Autodesk Fusion 360 part; units mm, degrees
(part 3 of 3)
sketch "Sketch2" plane through (0, 0, 0) normal (0, 0, 1) x (1, 0, 0)
  line L0 (0, 75.1711) -> (0, -79.242) construction
  circle A0 centre (30, 30) radius 2
  circle A1 centre (30, -30) radius 2
  circle A2 centre (15.25, 15.25) radius 1.6
  circle A3 centre (15.25, -15.25) radius 1.6
  circle A4 centre (0, -23) radius 6.5
  circle A5 centre (15.25, -31.25) radius 1.6
  line L1 (0, 0) -> (20.75, 0) construction
  line L2 (38.1, 30) -> (0, 30) construction
  circle A6 centre (30, 30) radius 8
  line L3 (35.6569, 24.3431) -> (27.4225, 16.1088)
  line L4 (35.6569, 24.3431) -> (45.9903, 24.3431) construction
  circle A7 centre (30, -30) radius 8
  line L5 (35.6569, -24.3431) -> (27.4225, -16.1088)
  line L6 (35.6569, -24.3431) -> (71.3243, -24.3431) construction
  arc A8 (27.4225, 16.1088) -> (27.4225, -16.1088) centre (43.5312, 0) ccw
  line L7 (17.65, 71.4902) -> (17.65, -40.3362) construction
  arc A9 (17.65, 40.3362) -> (25.2812, 36.4601) centre (22.45, 40.3362) ccw
  line L8 (0, -29.5) -> (0, -61) construction
  circle A10 centre (13.5, -61.45) radius 1.6
  line L9 (1.4087, -40.0557) -> (4.9594, -49.762)
  line L10 (4.7762, -51.1421) -> (1.2256, -56.1739)
  circle A11 centre (10.15, -39.65) radius 1.6
  circle A12 centre (10.15, -46.2) radius 1.6
  circle A13 centre (10.15, -52.75) radius 1.6
  line L11 (17.05, 0) -> (17.05, 11.5) construction
  line L12 (16, 10.45) -> (16, -10.45)
  arc A14 (16, -10.45) -> (18.1, -10.45) centre (17.05, -10.45) ccw
  line L13 (18.1, -10.45) -> (18.1, 10.45)
  arc A15 (18.1, 10.45) -> (16, 10.45) centre (17.05, 10.45) ccw
  line L14 (17.05, 11.5) -> (17.05, -11.5) construction
  line L15 (0, 36.5) -> (4.1, 36.5)
  line L16 (6.6, 39) -> (6.6, 50.3)
  line L17 (4.1, 52.8) -> (0, 52.8)
  line L18 (0, 52.8) -> (0, 36.5)
  arc A16 (6.6, 50.3) -> (4.1, 52.8) centre (4.1, 50.3) ccw
  arc A17 (4.1, 36.5) -> (6.6, 39) centre (4.1, 39) ccw
  arc A18 (25.2812, -36.4601) -> (17.65, -40.3362) centre (22.45, -40.3362) ccw
  circle A19 centre (13.5, -61.45) radius 4
  line L19 (17.65, -40.3362) -> (17.4999, -61.4784)
  arc A20 (11.9967, -65.1568) -> (4.58, -65.8955) centre (8.99, -72.5703) ccw
  circle A21 centre (12.2, 31.25) radius 1.6
  circle A22 centre (10, 45.75) radius 1.6
  circle A23 centre (10, 52.3) radius 1.6
  circle A24 centre (10, 58.85) radius 1.6
  circle A25 centre (13.5, 67.95) radius 1.6
  circle A26 centre (13.5, 67.95) radius 4.15
  line L20 (17.65, 67.95) -> (17.65, 40.3362)
  line L21 (0, 64.8) -> (6.85, 64.8)
  line L22 (9.35, 67.3) -> (9.35, 67.95)
  arc A27 (6.85, 64.8) -> (9.35, 67.3) centre (6.85, 67.3) ccw
  line L23 (14.15, 62.15) -> (14.15, 56.45)
  arc A28 (14.15, 56.45) -> (15.95, 56.45) centre (15.05, 56.45) ccw
  line L24 (15.95, 56.45) -> (15.95, 62.15)
  arc A29 (15.95, 62.15) -> (14.15, 62.15) centre (15.05, 62.15) ccw
  line L25 (15.05, 62.15) -> (15.05, 56.45) construction
  line L26 (0.6422, 23.9043) -> (5.9006, 26.3955)
  line L27 (0.9309, 18.9369) -> (7.3689, 24.0325)
  arc A30 (7.3689, 24.0325) -> (5.9006, 26.3955) centre (6.5, 25.1303) ccw
  arc A31 (-18.1, -10.45) -> (-16, -10.45) centre (-17.05, -10.45) ccw
  line L28 (-4.7762, -51.1421) -> (-1.2256, -56.1739)
  line L29 (-17.65, -40.3362) -> (-17.4999, -61.4784)
  circle A32 centre (-10.15, -52.75) radius 1.6
  circle A33 centre (-15.25, -15.25) radius 1.6
  circle A34 centre (-10.15, -39.65) radius 1.6
  circle A35 centre (-30, -30) radius 2
  circle A36 centre (-13.5, -61.45) radius 4
  circle A37 centre (-10.15, -46.2) radius 1.6
  line L30 (-35.6569, -24.3431) -> (-71.3243, -24.3431) construction
  line L31 (-1.4087, -40.0557) -> (-4.9594, -49.762)
  line L32 (-16, 10.45) -> (-16, -10.45)
  line L33 (-35.6569, -24.3431) -> (-27.4225, -16.1088)
  arc A38 (-4.58, -65.8955) -> (-11.9967, -65.1568) centre (-8.99, -72.5703) ccw
  arc A39 (-17.65, -40.3362) -> (-25.2812, -36.4601) centre (-22.45, -40.3362) ccw
  circle A40 centre (-13.5, -61.45) radius 1.6
  line L34 (0, -29.5) -> (0, -61) construction
  circle A41 centre (-30, -30) radius 8
  circle A42 centre (-15.25, -31.25) radius 1.6
  circle A43 centre (-13.5, 67.95) radius 1.6
  arc A44 (-25.2813, 36.4601) -> (-17.65, 40.3362) centre (-22.45, 40.3362) ccw
  line L35 (-15.95, 56.45) -> (-15.95, 62.15)
  line L36 (-14.15, 62.15) -> (-14.15, 56.45)
  line L37 (-4.1, 52.8) -> (0, 52.8)
  circle A45 centre (-15.25, 15.25) radius 1.6
  line L38 (-6.6, 39) -> (-6.6, 50.3)
  line L39 (-17.05, 11.5) -> (-17.05, -11.5) construction
  circle A46 centre (-10, 45.75) radius 1.6
  arc A47 (-4.1, 52.8) -> (-6.6, 50.3) centre (-4.1, 50.3) ccw
  circle A48 centre (-13.5, 67.95) radius 4.15
  line L40 (0, 64.8) -> (-6.85, 64.8)
  line L41 (-17.05, 0) -> (-17.05, 11.5) construction
  line L42 (-15.05, 62.15) -> (-15.05, 56.45) construction
  circle A49 centre (-12.2, 31.25) radius 1.6
  circle A50 centre (-10, 58.85) radius 1.6
  arc A51 (-14.15, 62.15) -> (-15.95, 62.15) centre (-15.05, 62.15) ccw
  line L43 (-0.6422, 23.9043) -> (-5.9006, 26.3955)
  line L44 (0, 52.8) -> (0, 36.5)
  circle A52 centre (-30, 30) radius 8
  arc A53 (-6.6, 39) -> (-4.1, 36.5) centre (-4.1, 39) ccw
  line L45 (-35.6569, 24.3431) -> (-27.4225, 16.1088)
  line L46 (-17.65, 67.95) -> (-17.65, 40.3362)
  line L47 (-0.9309, 18.9369) -> (-7.3689, 24.0325)
  arc A54 (-5.9006, 26.3955) -> (-7.3689, 24.0325) centre (-6.5, 25.1303) ccw
  circle A55 centre (-10, 52.3) radius 1.6
  arc A56 (-16, 10.45) -> (-18.1, 10.45) centre (-17.05, 10.45) ccw
  circle A57 centre (-30, 30) radius 2
  line L48 (-18.1, -10.45) -> (-18.1, 10.45)
  arc A58 (-15.95, 56.45) -> (-14.15, 56.45) centre (-15.05, 56.45) ccw
  arc A59 (-9.35, 67.3) -> (-6.85, 64.8) centre (-6.85, 67.3) ccw
  line L49 (-9.35, 67.3) -> (-9.35, 67.95)
  line L50 (-35.6569, 24.3431) -> (-45.9903, 24.3431) construction
  line L51 (0, 0) -> (-20.75, 0) construction
  arc A60 (-27.4225, -16.1088) -> (-27.4225, 16.1088) centre (-43.5312, 0) ccw
  line L52 (0, 36.5) -> (-4.1, 36.5)
  line L53 (-17.65, 71.4902) -> (-17.65, -40.3362) construction
  line L54 (-38.1, 30) -> (0, 30) construction
  arc A61 (-0.6422, 23.9043) -> (0.6422, 23.9043) centre (0, 25.2598) ccw
  arc A62 (-0.9309, 18.9369) -> (0.9309, 18.9369) centre (0, 20.113) ccw
  arc A63 (1.4087, -40.0557) -> (-1.4087, -40.0557) centre (0, -40.571) ccw
  arc A64 (-1.2256, -56.1739) -> (1.2256, -56.1739) centre (0, -55.3091) ccw
  arc A65 (4.7762, -51.1421) -> (4.9594, -49.762) centre (3.5507, -50.2773) ccw
  arc A66 (-4.9594, -49.762) -> (-4.7762, -51.1421) centre (-3.5507, -50.2773) ccw
  line L55 (3.0607, 1.0607) -> (7.4393, 5.4393)
  line L56 (2, 0) -> (13.2991, 0) construction
  line L57 (10, 4.3787) -> (10, -4.3787)
  line L58 (3.0607, -1.0607) -> (7.4393, -5.4393)
  line L59 (2, 0) -> (13.2991, 0) construction
  arc A67 (10, 4.3787) -> (7.4393, 5.4393) centre (8.5, 4.3787) ccw
  arc A68 (3.0607, 1.0607) -> (3.0607, -1.0607) centre (4.1213, 0) ccw
  arc A69 (7.4393, -5.4393) -> (10, -4.3787) centre (8.5, -4.3787) ccw
  arc A70 (5.4393, 7.4393) -> (4.3787, 10) centre (4.3787, 8.5) ccw
  line L60 (-4.3787, 10) -> (4.3787, 10)
  line L61 (1.0607, 3.0607) -> (5.4393, 7.4393)
  line L62 (-1.0607, 3.0607) -> (-5.4393, 7.4393)
  arc A71 (-1.0607, 3.0607) -> (1.0607, 3.0607) centre (0, 4.1213) ccw
  arc A72 (-4.3787, 10) -> (-5.4393, 7.4393) centre (-4.3787, 8.5) ccw
  arc A73 (-7.4393, 5.4393) -> (-10, 4.3787) centre (-8.5, 4.3787) ccw
  line L63 (-10, -4.3787) -> (-10, 4.3787)
  line L64 (-3.0607, 1.0607) -> (-7.4393, 5.4393)
  line L65 (-3.0607, -1.0607) -> (-7.4393, -5.4393)
  arc A74 (-3.0607, -1.0607) -> (-3.0607, 1.0607) centre (-4.1213, 0) ccw
  arc A75 (-10, -4.3787) -> (-7.4393, -5.4393) centre (-8.5, -4.3787) ccw
  arc A76 (-5.4393, -7.4393) -> (-4.3787, -10) centre (-4.3787, -8.5) ccw
  line L66 (4.3787, -10) -> (-4.3787, -10)
  line L67 (-1.0607, -3.0607) -> (-5.4393, -7.4393)
  line L68 (1.0607, -3.0607) -> (5.4393, -7.4393)
  arc A77 (1.0607, -3.0607) -> (-1.0607, -3.0607) centre (0, -4.1213) ccw
  arc A78 (4.3787, -10) -> (5.4393, -7.4393) centre (4.3787, -8.5) ccw
  arc A79 (3.8096, -65.4061) -> (-3.8096, -65.4061) centre (0, -64.85) ccw
  arc A80 (-4.58, -65.8955) -> (-3.8096, -65.4061) centre (-4.3044, -65.4784) ccw
  arc A81 (3.8096, -65.4061) -> (4.58, -65.8955) centre (4.3044, -65.4784) ccw
  point P0 (5.2293, -50.5)
  point P1 (6.6, 36.5)
  point P2 (0, 18.2)
  point P3 (0, -23)
  point P4 (0, -79.242)
  point P5 (0, -64.85)
  point P6 (0, 18.2)
  point P7 (-6.6, 36.5)
  point P8 (0, 23.6)
  point P9 (0, 75.1711)
  point P10 (0, 2)
  point P11 (-2, 0)
  point P12 (0, -2)
  dimension "d1" = 4
  dimension "d2" = 30
  dimension "d3" = 30
  dimension "d4" = 30
  dimension "d5" = 30
  dimension "d6" = 3.2
  dimension "d7" = 15.25
  dimension "d8" = 15.25
  dimension "d9" = 15.25
  dimension "d10" = 15.25
  dimension "d11" = 7.7
  dimension "d12" = 13
  dimension "d13" = 23
  dimension "d14" = 15.25
  dimension "d15" = 16
  dimension "d16" = 20.75
  dimension "d17" = 38.1
  dimension "d18" = 16
  dimension "d19" = 135
  dimension "d20" = 16
  dimension "d21" = 135
  dimension "d23" = 17.65
  dimension "d24" = 4.8
  dimension "d25" = 31.5
  dimension "d26" = 13.5
  dimension "d27" = 30.2
  dimension "d28" = 8.4
  dimension "d29" = 5.1
  dimension "d32" = 0
  dimension "d33" = -13.1
  dimension "d34" = 11.5
  dimension "d35" = 2.1
  dimension "d36" = 16
  dimension "d37" = 23
  dimension "d38" = 6.6
  dimension "d39" = 16.3
  dimension "d40" = 2.5
  dimension "d41" = 36.5
  dimension "d42" = 4.8
  dimension "d43" = 8
  dimension "d45" = 8
  dimension "d46" = 16
  dimension "d48" = 50.5
  dimension "d49" = 14.5
  dimension "d50" = 10
  dimension "d53" = 0
  dimension "d54" = 13.1
  dimension "d55" = 12.2
  dimension "d56" = 13.5
  dimension "d57" = 52.7
  dimension "d58" = 12
  dimension "d59" = 2.5
  dimension "d60" = 1.8
  dimension "d61" = 5.7
  dimension "d62" = 1.7
  dimension "d63" = 5.8
  dimension "d64" = 18.2
  dimension "d65" = 1.4
  dimension "d66" = 6.5
  dimension "d67" = 5.4
  dimension "d68" = 1.5
  dimension "d69" = 1.5
  dimension "d70" = 1.5
  dimension "d71" = 45
  dimension "d72" = 45
  dimension "d73" = 2
  dimension "d74" = 8
  dimension "d75" = 1.5
  dimension "d77" = 360
  dimension "d80" = 0.5
  constraint vertical L0
  constraint equal A0 A1
  constraint equal A2 A3
  constraint coincident L0 P5
  constraint coincident L0 P3
  constraint equal A3 A5
  constraint coincident L1.start L51.start
  constraint perpendicular L0 L1
  constraint coincident L0 L2.end
  constraint perpendicular L0 L2
  constraint coincident A0.centre L2
  constraint concentric A0 A6
  constraint horizontal L4
  constraint coincident A6 L3.start
  constraint tangent A6 L3
  constraint concentric A1 A7
  constraint horizontal L6
  constraint coincident A7 L5.start
  constraint tangent A7 L5
  constraint tangent L3 A8
  constraint tangent L5 A8
  constraint vertical L7
  constraint coincident L1.end A8
  constraint coincident L7 A9.start
  constraint coincident A6 A9.end
  constraint tangent A6 A9
  constraint tangent L7 A9
  constraint coincident A4 L8.start
  constraint coincident L8.end A79
  constraint parallel L0 L8
  constraint coincident L0 L8.end
  constraint equal A5 A10
  constraint equal A5 A11
  constraint coincident L1 L11.start
  constraint perpendicular L1 L11
  constraint tangent L12 A14
  constraint tangent A14 L13
  constraint parallel L12 L13
  constraint tangent L13 A15
  constraint tangent L12 A15
  constraint midpoint L11.end A15
  constraint midpoint A14 L14.end
  constraint parallel L7 L14
  constraint horizontal L15
  constraint vertical L16
  constraint horizontal L17
  constraint vertical L18
  constraint coincident L0 L15.start
  constraint tangent L16 A16
  constraint tangent L17 A16
  constraint coincident P1 L15
  constraint coincident P1 L16
  constraint tangent L15 A17
  constraint tangent L16 A17
  constraint equal A16 A17
  constraint tangent L7 A18
  constraint coincident A7 A18.start
  constraint tangent A7 A18
  constraint concentric A10 A19
  constraint coincident A19 L19.end
  constraint tangent A19 L19
  constraint tangent A19 A20
  constraint coincident A19 A20.start
  constraint tangent A20 A79
  constraint equal A2 A21
  constraint equal A21 A22
  constraint equal A24 A25
  constraint concentric A25 A26
  constraint tangent L7 A26
  constraint coincident A26 L20.start
  constraint tangent A9 L20
  constraint coincident L0 L21.start
  constraint perpendicular L0 L21
  constraint coincident A26 L22.end
  constraint vertical L22
  constraint tangent A26 L22
  constraint tangent L21 A27
  constraint tangent L22 A27
  constraint tangent L23 A28
  constraint tangent A28 L24
  constraint parallel L23 L24
  constraint tangent L24 A29
  constraint tangent L23 A29
  constraint perpendicular L21 L25
  constraint coincident L0 P6
  constraint tangent L26 A30
  constraint tangent L27 A30
  constraint symmetric L1.start L0 L51.start
  constraint symmetric P9 L0 L0.start
  constraint symmetric P4 L0 L0.end
  constraint symmetric L0 A0 A57
  constraint symmetric L0 A1 A35
  constraint symmetric L0 A2 A45
  constraint symmetric L0 A3 A33
  constraint symmetric L0 P5 A79.centre
  constraint symmetric L0 P3 A4.centre
  constraint symmetric L0 A5 A42
  constraint symmetric L0 L1.start L51.start
  constraint symmetric L0 L1.end L51.end
  constraint symmetric L0 L2.start L54.start
  constraint symmetric L0 L2.end L54.end
  constraint symmetric L0 A6 A52
  constraint symmetric L0 L3.start L45.start
  constraint symmetric L0 L4.end L50.end
  constraint symmetric L0 A7 A41
  constraint symmetric L0 L5.start L30.start
  constraint symmetric L0 L6.end L30.end
  constraint symmetric L0 L3.end L45.end
  constraint symmetric L0 L5.end L33.end
  constraint symmetric L0 A8 A60
  constraint symmetric L0 L7.start L53.start
  constraint symmetric L0 A9.start A44.end
  constraint symmetric L0 A9 A44
  constraint symmetric L0 L8.start L34.start
  constraint symmetric L0 L8.end L34.end
  constraint symmetric L0 A10 A40
  constraint symmetric L0 A11 A34
  constraint symmetric L0 A12 A37
  constraint symmetric L0 A13 A32
  constraint symmetric L0 L11.start L41.start
  constraint symmetric L0 L11.end L39.start
  constraint symmetric L0 L12.start L32.start
  constraint symmetric L0 L12.end A31.end
  constraint symmetric L0 A14.end A31.start
  constraint symmetric L0 L13.end A56.end
  constraint symmetric L0 A14 A31
  constraint symmetric L0 A15 A56
  constraint symmetric L0 L14.end L39.end
  constraint symmetric L0 L15.start L18.end
  constraint symmetric L0 P1 P7
  constraint symmetric L0 L17.end L18.start
  constraint symmetric L0 L16.end L38.end
  constraint symmetric L0 L17.start L37.start
  constraint symmetric L0 A16 A47
  constraint symmetric L0 L15.end A53.end
  constraint symmetric L0 L16.start L38.start
  constraint symmetric L0 A17 A53
  constraint symmetric L0 A18.start A39.end
  constraint symmetric L0 L7.end L29.start
  constraint symmetric L0 A18 A39
  constraint symmetric L0 A19 A36
  constraint symmetric L0 L19.end L29.end
  constraint symmetric L0 A20.start A38.end
  constraint symmetric L0 A20 A38
  constraint symmetric L0 A21 A49
  constraint symmetric L0 A22 A46
  constraint symmetric L0 A23 A55
  constraint symmetric L0 A24 A50
  constraint symmetric L0 A25 A43
  constraint symmetric L0 A26 A48
  constraint symmetric L0 L20.start L46.start
  constraint symmetric L0 L21.start L40.start
  constraint symmetric L0 L22.end L49.end
  constraint symmetric L0 L21.end L40.end
  constraint symmetric L0 L22.start A59.start
  constraint symmetric L0 A27 A59
  constraint symmetric L0 L23.start L36.start
  constraint symmetric L0 L23.end L36.end
  constraint symmetric L0 A28.end L35.start
  constraint symmetric L0 L24.end L35.end
  constraint symmetric L0 A28 A58
  constraint symmetric L0 A29 A51
  constraint symmetric L0 P6 P2
  constraint symmetric L0 L26.end L43.end
  constraint symmetric L0 L27.end L47.end
  constraint symmetric L0 A30 A54
  constraint coincident P8 L43
  constraint tangent L26 A61
  constraint tangent L43 A61
  constraint coincident P6 L27
  constraint coincident P6 L47
  constraint tangent L27 A62
  constraint tangent L47 A62
  constraint equal A61 A62
  constraint tangent L9 A63
  constraint tangent L31 A63
  constraint tangent L28 A64
  constraint tangent L10 A64
  constraint coincident P0 L9
  constraint coincident P0 L10
  constraint tangent L9 A65
  constraint tangent L10 A65
  constraint equal A64 A65
  constraint tangent L31 A66
  constraint tangent L28 A66
  constraint equal A64 A66
  constraint horizontal L56
  constraint coincident L1 L56.start
  constraint perpendicular L1 L57
  constraint horizontal L59
  constraint tangent L55 A67
  constraint tangent L57 A67
  constraint coincident L56.start L58
  constraint coincident L56.start L55
  constraint tangent L58 A68
  constraint tangent L55 A68
  constraint equal A67 A68
  constraint tangent L58 A69
  constraint tangent L57 A69
  constraint equal A67 A69
  constraint tangent A79 A80
  constraint tangent A38 A80
  constraint tangent A79 A81
  constraint tangent A20 A81
  constraint equal A80 A81
  measures "d1" diameter of A0
  measures "d2" distance of L0 A0.centre
  measures "d3" vertical distance of L1.start A0.centre
  measures "d4" distance of L0 A1.centre
  measures "d5" vertical distance of L1.start A1.centre
  measures "d6" diameter of A2
  measures "d7" distance of L0 A2.centre
  measures "d8" vertical distance of L1.start A2.centre
  measures "d9" distance of L0 A3.centre
  measures "d10" vertical distance of L1.start A3.centre
  measures "d11" diameter of A79
  measures "d12" diameter of A4
  measures "d13" distance of L1.start P3
  measures "d14" distance of L0 A5.centre
  measures "d15" distance of A3.centre A5.centre
  measures "d16" distance of L1.start L1.end
  measures "d17" distance of L2.start L2.end
  measures "d18" diameter of A6
  measures "d19" angle of L3 L4
  measures "d20" diameter of A7
  measures "d21" angle of L5 L6
  measures "d23" distance of L0 L7
  measures "d24" radius of A9
  measures "d25" distance of L8.start L8.end
  measures "d26" distance of L0 A10.centre
  measures "d27" vertical distance of A5.centre A10.centre
  measures "d28" vertical distance of A5.centre A11.centre
  measures "d29" horizontal distance of A5.centre A11.centre
  measures "d34" distance of L11.start L11.end
  measures "d35" diameter of A14
  measures "d36" distance of L1.start L12
  measures "d37" distance of L11.end L14.end
  measures "d38" distance of L15.start P1
  measures "d39" distance of L15.start L17.end
  measures "d40" radius of A16
  measures "d41" distance of L1.start L15.start
  measures "d42" radius of A18
  measures "d43" diameter of A19
  measures "d45" radius of A20
  measures "d46" vertical distance of A2.centre A21.centre
  measures "d48" vertical distance of L1.start P0
  measures "d49" vertical distance of A21.centre A22.centre
  measures "d50" distance of L0 A22.centre
  measures "d55" distance of L0 A21.centre
  measures "d56" distance of L0 A25.centre
  measures "d57" vertical distance of A2.centre A25.centre
  measures "d58" distance of L17 L21
  measures "d59" radius of A27
  measures "d60" distance of L23 L24
  measures "d61" distance of A29.centre A28.centre
  measures "d62" distance of L7 L24
  measures "d63" vertical distance of A25.centre A29.centre
  measures "d64" distance of L1.start P6
  measures "d65" radius of A30
  measures "d66" distance of L0 A30.centre
  measures "d67" distance of P6 P8
  measures "d68" radius of A61
  measures "d69" radius of A63
  measures "d70" radius of A64
  measures "d71" angle of L55 L56
  measures "d72" angle of L58 L59
  measures "d73" distance of L1.start L56.start
  measures "d74" distance of L56.start L57
  measures "d75" radius of A67
  measures "d80" radius of A80
extrude "Extrude1" add sketch "Sketch2" along normal blind 2
equation "d2 = ( 60 / 2 ) * 1 mm"
equation "d3 = d2"
equation "d4 = d2"
equation "d5 = d3"
equation "d7 = ( 30.5 / 2 ) * 1 mm"
equation "d8 = d7"
equation "d9 = d7"
equation "d10 = d8"
equation "d14 = d9"
equation "d16 = ( 41.5 / 2 ) * 1 mm"
equation "d17 = ( 76.2 / 2 ) * 1 mm"
equation "d20 = d18"
equation "d23 = ( 35.3 / 2 ) * 1 mm"
equation "d26 = ( 27 / 2 ) * 1 mm"
equation "d34 = ( 23 / 2 ) * 1 mm"
equation "d38 = ( 13.2 / 2 ) * 1 mm"
equation "d42 = d24"
equation "d50 = ( 20 / 2 ) * 1 mm"
equation "d55 = ( 24.4 / 2 ) * 1 mm"
equation "d56 = ( 27 / 2 ) * 1 mm"
equation "d61 = 7.5 mm - 1.8 mm"

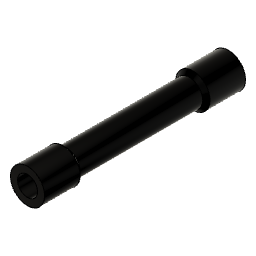
design "standoff"
Autodesk Fusion 360 part; units mm, degrees
sketch "Sketch1" plane through (0, 0, 0) normal (0, 1, 0) x (1, 0, 0)
  line L0 (0, 0) -> (0, 30)
  line L1 (0, 30) -> (2.55, 30)
  line L2 (2.55, 30) -> (2.55, 24.7)
  line L3 (0, 0) -> (2.55, 0)
  line L4 (2.55, 0) -> (2.55, 5.3)
  line L5 (2, 0) -> (2, 30)
  line L6 (2.55, 24.7) -> (2, 24.15)
  line L7 (2.55, 24.7) -> (3.3278, 24.7) construction
  line L8 (2.55, 5.3) -> (2, 5.85)
  dimension "d1" = 30
  dimension "d2" = 2.55
  dimension "d3" = 5.3
  dimension "d4" = 2.55
  dimension "d5" = 5.3
  dimension "d6" = 2
  dimension "d7" = 135
  constraint coincident L0.start L3.start
  constraint vertical L0
  constraint perpendicular L0 L1
  constraint perpendicular L1 L2
  constraint perpendicular L0 L3
  constraint perpendicular L3 L4
  constraint horizontal L7
  constraint coincident L5 L6.end
  constraint coincident L5 L8.end
  constraint perpendicular L6 L8
  measures "d1" distance of L0.start L0.end
  measures "d2" distance of L0.end L1.end
  measures "d3" distance of L1.end L2.end
  measures "d4" distance of L0.start L3.end
  measures "d5" distance of L3.end L4.end
  measures "d7" angle of L6 L7
revolve "Revolve1" add sketch "Sketch1" angle 360 about axis through (0, 0, 0) along (0, 0, -1)
sketch "Sketch2" plane through (0, 0, -30) normal (0, 0, -1) x (-1, 0, 0)
  circle A0 centre (0, 0) radius 2.55
  circle A1 centre (0, 0) radius 1.5
  dimension "d9" = 3
  constraint concentric A0 A1
  measures "d9" diameter of A1
extrude "Extrude1" cut sketch "Sketch2" against normal up to surface (30 mm away) contours A1
equation "d2 = ( 5.1 / 2 ) * 1 mm"
equation "d4 = d2"
equation "d5 = d3"
